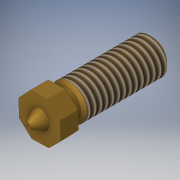
# Autodesk Inventor part: E3D-v6 Volcano Nozzle
Saved by Autodesk Inventor 2018.2 (Build 222227000, 227)
## iProperties
Created: 2018-02-27
Part Number: E3D-v6 Volcano Nozzle
Material: Messing, weicher Gelbton
Document SubType Name: Modeling
Designer: Till
Density: 8.47 g/cm^3
Appearance: Messing - satiniert
Author: Till
Autodesk Inventor part; units mm, degrees
ref_plane "YZ Plane" through (0, 0, 0) normal (1, 0, 0) x (0, 1, 0)
ref_plane "XZ Plane" through (0, 0, 0) normal (0, 1, 0) x (-1, 0, 0)
ref_plane "XY Plane" through (0, 0, 0) normal (0, 0, 1) x (1, 0, 0)
sketch "Skizze1" plane through (0, 0, 0) normal (0, 0, 1) x (1, 0, 0)
  line L0 (0.2, 0) -> (0.5, 0)
  line L1 (0.2, 0) -> (0.5, 0) construction
  line L2 (0.5, 0) -> (1.6547, 2)
  line L3 (1.6547, 2) -> (3.5, 2)
  line L4 (3.5, 2) -> (3.5, 5)
  line L5 (3.5, 5) -> (2.5, 5)
  line L6 (2.5, 5) -> (2.5, 6.5)
  line L7 (2.5, 6.5) -> (3, 6.5)
  line L8 (3, 6.5) -> (3, 21)
  line L9 (3, 21) -> (1, 21)
  line L10 (1, 21) -> (1, 1.9856)
  line L11 (0.2, 0) -> (0.2, 0.6)
  line L12 (0.2, 0.6) -> (1, 1.9856)
  line L13 (0, -4.2) -> (0, 25.2) projected
  point P0 (0, 0)
  dimension "d4" = 90
  dimension "d6" = 1
  dimension "d7" = 0.2
  dimension "d8" = 0
  dimension "d9" = 0.5
  dimension "d10" = 19
  dimension "d11" = 16
  dimension "d12" = 14.5
  dimension "d13" = 2.5
  dimension "d15" = 21
  dimension "d16" = 0.6
  dimension "d17" = 3.5
  dimension "d18" = 150
  dimension "d19" = 3
  constraints: 26 end point, 6 perpendicular, 2 horizontal, 1 collinear, 1 parallel, 1 vertical
  measures "d4" angle of L10 L9
  measures "d6" distance from line of L10 point (0, 0)
  measures "d7" distance of point (0, 0) L0.start
  measures "d8" distance from line of point (0, 0) L0
  measures "d9" distance of point (0, 0) L0.end
  measures "d10" distance between parallel lines of L9 L3
  measures "d11" distance between parallel lines of L5 L9
  measures "d12" distance between parallel lines of L9 L7
  measures "d13" distance from line of point (0, 0) L6
  measures "d15" distance between parallel lines of L9 L0
  measures "d16" distance of L0.start L11.end
  measures "d17" distance from line of point (0, 0) L4
  measures "d18" angle of L11 L12
  measures "d19" distance from line of point (0, 0) L8
revolve "Umdrehung1" add sketch "Skizze1" angle 360 about axis through (0, -10, 0) along (0, 1, 0)
sketch "Skizze2" plane through (0, 2, 0) normal (0, -1, 0) x (1, 0, 0)
  circle A0 centre (0, 0) radius 0.2 projected
  line L0 (3.5412, -1.346) -> (1.5522, -3.4558)
  line L1 (1.5522, -3.4558) -> (-1.346, -3.5412)
  line L2 (-1.346, -3.5412) -> (-3.4558, -1.5522)
  line L3 (-3.4558, -1.5522) -> (-3.5412, 1.346)
  line L4 (-3.5412, 1.346) -> (-1.5522, 3.4558)
  line L5 (-1.5522, 3.4558) -> (1.346, 3.5412)
  line L6 (1.346, 3.5412) -> (3.4558, 1.5522)
  line L7 (3.4558, 1.5522) -> (3.5412, -1.346)
  circle A1 centre (0, 0) radius 1.6547
  dimension "d21" = 7
  constraints: 16 end point, 2 coincident, 1 centre point, 17 other
  measures "d21" distance between parallel lines of L3 L7
extrude "Extrusion2" add sketch "Skizze2" against normal up to surface (3 mm away) contours L0 L1 L2 L3 L4 L5 L6 L7
thread "Gewinde1" size "M6x1" class "6g" standard "ANSI Metric M Profile" full length
chamfer "Fase1" distance 0.5 angle 45 2 edges at (-3, 6.5, 0) (-3, 21, 0)
